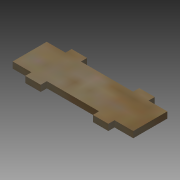
# Autodesk Inventor part: front(magi)
Saved by Autodesk Inventor 2016 (Build 200138000, 138)
## iProperties
Created: 2015-10-07
Part Number: front(magi)
Material: Generic
Document SubType Name: Modeling
Designer: Haukur
Density: 1 g/cm^3
Appearance: Plywood - Weathered
Author: Haukur
Autodesk Inventor part; units mm, degrees
ref_plane "YZ Plane" through (0, 0, 0) normal (1, 0, 0) x (0, 1, 0)
ref_plane "XZ Plane" through (0, 0, 0) normal (0, 1, 0) x (-1, 0, 0)
ref_plane "XY Plane" through (0, 0, 0) normal (0, 0, 1) x (1, 0, 0)
sketch "Sketch1" plane through (0, 0, 0) normal (0, 0, 1) x (1, 0, 0)
  line L0 (0, 4) -> (0, 26)
  line L1 (0, 26) -> (12.101, 26)
  line L2 (12.101, 26) -> (12.101, 30)
  line L3 (12.101, 30) -> (22.101, 30)
  line L4 (22.101, 30) -> (22.101, 26)
  line L5 (22.101, 26) -> (55.782, 26)
  line L6 (55.782, 26) -> (55.782, 30)
  line L7 (55.782, 30) -> (65.782, 30)
  line L8 (65.782, 30) -> (65.782, 26)
  line L9 (65.782, 26) -> (77.883, 26)
  line L10 (77.883, 26) -> (77.883, 4)
  line L11 (77.883, 4) -> (65.782, 4)
  line L12 (65.782, 4) -> (65.782, 0)
  line L13 (65.782, 0) -> (55.782, 0)
  line L14 (55.782, 0) -> (55.782, 4)
  line L15 (55.782, 4) -> (22.101, 4)
  line L16 (22.101, 4) -> (22.101, 0)
  line L17 (22.101, 0) -> (12.101, 0)
  line L18 (12.101, 0) -> (12.101, 4)
  line L19 (12.101, 4) -> (0, 4)
  point P0 (0, 0)
  dimension "d0" = 22
  dimension "d1" = 12.101
  dimension "d2" = 4
  dimension "d3" = 10
  dimension "d4" = 33.681
  dimension "d5" = 10
  dimension "d6" = 12.101
  constraints: 40 end point, 13 perpendicular, 12 point on line, 1 horizontal, 1 vertical
  measures "d0" distance of L0.start L0.end
  measures "d1" distance of L0.end L1.end
  measures "d2" distance of L1.end L2.end
  measures "d3" distance of L2.end L3.end
  measures "d4" distance of L4.end L5.end
  measures "d5" distance of L6.end L7.end
  measures "d6" distance of L8.end L9.end
extrude "Extrusion1" add sketch "Sketch1" along normal blind 4
body "Solid1"
